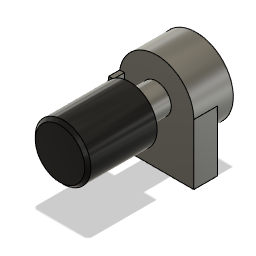
LoTec Vent CON2 (Autodesk Fusion 360 archive; units mm, degrees)
design "POT PRESSURE"
Autodesk Fusion 360 part; units mm, degrees
sketch "Sketch1" plane through (0, 0, 0) normal (0, 0, 1) x (1, 0, 0)
  circle A0 centre (0, 0) radius 3.36
  line L0 (-8.3921, 1.35) -> (-7.31, 1.35)
  line L1 (-7.31, 1.35) -> (-7.31, -1.35)
  line L2 (-7.31, -1.35) -> (-8.3921, -1.35)
  circle A1 centre (0, 0) radius 8.5
  line L3 (-8.5, -0.0037) -> (-8.5, -13.82)
  line L4 (8.5, 0) -> (8.5, -13.82)
  line L5 (8.5, -13.82) -> (-8.5, -13.82)
  dimension "d1" = 6.72
  dimension "d4" = 7.31
  dimension "d5" = 17
  dimension "d6" = 1.35
  dimension "d7" = 13.82
  constraint coincident A0.centre A1.centre
  constraint horizontal L0
  constraint vertical L1
  constraint horizontal L2
  constraint coincident A1 L2.end
  constraint coincident A1 L0.start
  constraint coincident A1 L3.start
  constraint perpendicular L2 L3
  constraint coincident A1 L4.start
  constraint tangent A1 L4
  constraint parallel L3 L4
  constraint perpendicular L4 L5
  measures "d1" diameter of A0
  measures "d4" distance of A0.centre L1
  measures "d5" diameter of A1
  measures "d6" distance of A0.centre L0
  measures "d7" distance of A0.centre L5
extrude "Extrude1" add sketch "Sketch1" along normal blind 20 contours A0 makes body 1
extrude "Extrude2" add sketch "Sketch1" against normal blind 9 contours A0 | L0 L1 L2 A1 | L0 L1 L2 A1 bodies 1
extrude "Extrude3" add sketch "Sketch1" along normal blind 2.5 contours L0 L1 L2 A1 picked at (-7.7067, -0.0012) bodies 1
sketch "Sketch2" plane through (0, 0, 20) normal (0, 0, 1) x (1, 0, 0)
  circle A0 centre (0, 0) radius 3.36
  circle A1 centre (0, 0) radius 6.33
  dimension "d14" = 12.66
  constraint concentric A0 A1
  measures "d14" diameter of A1
extrude "Extrude4" add sketch "Sketch2" along normal blind 2 and the other way blind 13.8 separate body contours A0 | A1 makes body 2
chamfer "Chamfer1" distance 0.691 angle 45 1 edges at (-5.9016, -2.289, 22) on bodies 2
extrude "Extrude5" add sketch "Sketch1" against normal blind 5.389 contours A1 L3 L4 L5 bodies 1

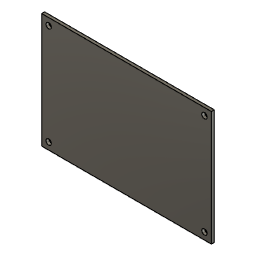
design "circuit board"
Autodesk Fusion 360 part; units mm, degrees
sketch "Sketch1" plane through (0, 0, 0) normal (0, 0, 1) x (1, 0, 0)
  line L0 (46.925, -31.75) -> (-46.925, -31.75)
  line L1 (-46.925, -31.75) -> (-46.925, 31.75)
  line L2 (-46.925, 31.75) -> (46.925, 31.75)
  line L3 (46.925, 31.75) -> (46.925, -31.75)
  line L4 (46.925, -31.75) -> (-46.925, 31.75) construction
  line L5 (-46.925, -31.75) -> (46.925, 31.75) construction
  line L6 (43.08, 27.835) -> (-43.08, 27.835)
  line L7 (-43.08, 27.835) -> (-43.08, -27.835)
  line L8 (-43.08, -27.835) -> (43.08, -27.835)
  line L9 (43.08, -27.835) -> (43.08, 27.835)
  line L10 (43.08, 27.835) -> (-43.08, -27.835) construction
  line L11 (-43.08, 27.835) -> (43.08, -27.835) construction
  circle A0 centre (-43.08, 27.835) radius 1.5
  circle A1 centre (43.08, 27.835) radius 1.5
  circle A2 centre (43.08, -27.835) radius 1.5
  circle A3 centre (-43.08, -27.835) radius 1.5
  dimension "d1" = 93.85
  dimension "d2" = 63.5
  dimension "d3" = 86.16
  dimension "d4" = 55.67
  dimension "d5" = 3
  dimension "d6" = 3
  dimension "d7" = 3
  dimension "d8" = 3
  constraint horizontal L0
  constraint perpendicular L0 L1
  constraint parallel L0 L2
  constraint parallel L1 L3
  constraint coincident L4 origin
  constraint coincident L5 origin
  constraint horizontal L6
  constraint perpendicular L6 L7
  constraint parallel L6 L8
  constraint parallel L7 L9
  constraint coincident L10 origin
  constraint coincident L11 origin
  constraint coincident L6.end L7.start
  constraint coincident L6.start L9.end
  constraint coincident L8.end L9.start
  constraint coincident L7.end L8.start
  measures "d1" distance of L1.end L2.end
  measures "d2" distance of L0.end L1.end
  measures "d3" distance of L7.end L8.end
  measures "d4" distance of L6.end L7.end
  measures "d5" diameter of A0
  measures "d6" diameter of A1
  measures "d7" diameter of A2
  measures "d8" diameter of A3
extrude "Extrude1" add sketch "Sketch1" along normal blind 1.6 contours L0 L1 L2 L3 | L6 L7 L8 L9 A0 A1 A2 A3

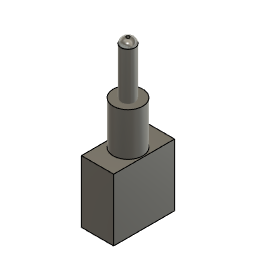
design "ON OFF ON SWITCH"
Autodesk Fusion 360 part; units mm, degrees
sketch "Sketch1" plane through (0, 0, 0) normal (0, 1, 0) x (1, 0, 0)
  circle A0 centre (0, 0) radius 3.095
  line L0 (3.375, 6.375) -> (-3.375, 6.375)
  line L1 (-3.375, 6.375) -> (-3.375, -6.375)
  line L2 (-3.375, -6.375) -> (3.375, -6.375)
  line L3 (3.375, -6.375) -> (3.375, 6.375)
  line L4 (3.375, 6.375) -> (-3.375, -6.375) construction
  line L5 (-3.375, 6.375) -> (3.375, -6.375) construction
  circle A1 centre (0, 0) radius 1.5
  dimension "d1" = 6.19
  dimension "d2" = 6.75
  dimension "d3" = 12.75
  dimension "d8" = 3
  constraint coincident A0.centre A1.centre
  constraint horizontal L0
  constraint perpendicular L0 L1
  constraint parallel L0 L2
  constraint parallel L1 L3
  constraint coincident L4 A0.centre
  constraint coincident L5 A0.centre
  measures "d1" diameter of A0
  measures "d2" distance of L1.end L2.end
  measures "d3" distance of L0.end L1.end
  measures "d8" diameter of A1
extrude "Extrude1" add sketch "Sketch1" along normal blind 9 contours A0 | A1 makes body 1
extrude "Extrude2" add sketch "Sketch1" against normal blind 13 contours A0 | L0 L1 L2 L3 | A1 bodies 1
extrude "Extrude3" add sketch "Sketch1" along normal blind 20 separate body contours A1 makes body 2
fillet "Fillet1" radius 1.182 1 edges at (-1.3985, 20, 0.5424) on bodies 2
